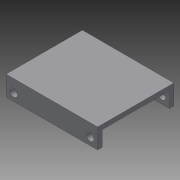
# Autodesk Inventor part: EE_Base-SquareBar-Rev3
Saved by Autodesk Inventor 2015 (Build 190159000, 159)
## iProperties
Created: 2017-01-10
Part Number: EE_Base-SquareBar-Rev3
Material: Generic
Document SubType Name: Modeling
Designer: Guy
Density: 1 g/cm^3
Appearance: Default
Author: Guy
Autodesk Inventor part; units mm, degrees
ref_plane "YZ Plane" through (0, 0, 0) normal (1, 0, 0) x (0, 1, 0)
ref_plane "XZ Plane" through (0, 0, 0) normal (0, 1, 0) x (-1, 0, 0)
ref_plane "XY Plane" through (0, 0, 0) normal (0, 0, 1) x (1, 0, 0)
sketch "Sketch1" plane through (0, 0, 0) normal (0, 0, 1) x (1, 0, 0)
  line L0 (0, 0) -> (60, 0)
  line L1 (60, 0) -> (60, 50)
  line L2 (60, 50) -> (0, 50)
  line L3 (0, 50) -> (0, 0)
  dimension "d0" = 60
  dimension "d1" = 50
  constraints: 8 end point, 2 parallel, 1 horizontal, 1 perpendicular
  measures "d0" distance of L2.end L1.end
  measures "d1" distance between parallel lines of L0 L2
extrude "Extrusion1" add sketch "Sketch1" along normal blind 3
sketch "Sketch2" plane through (0, 0, 0) normal (0, 0, -1) x (-1, 0, 0)
  line L0 (0, 0) -> (-60, 0) projected
  line L1 (0, 50) -> (0, 0) projected
  line L2 (-60, 50) -> (0, 50) projected
  line L3 (-60, 0) -> (-60, 50) projected
  line L4 (0, 0) -> (-60, 0)
  line L5 (-60, 0) -> (-60, 3)
  line L6 (-60, 3) -> (0, 3)
  line L7 (0, 3) -> (0, 0)
  line L8 (-60, 0) -> (-60, 50) projected
  line L9 (0, 50) -> (-60, 50)
  line L10 (-60, 50) -> (-60, 47)
  line L11 (-60, 47) -> (0, 47)
  line L12 (0, 47) -> (0, 50)
  dimension "d4" = 3
  dimension "d5" = 3
  constraints: 16 end point, 4 parallel, 2 horizontal, 2 perpendicular, 2 point on line
  measures "d4" distance between parallel lines of L6 L0
  measures "d5" distance between parallel lines of L2 L11
extrude "Extrusion2" add sketch "Sketch2" along normal blind 10 contours L0 L3 L6 L1 | L11 L3 L2 L1
sketch "Sketch3" plane through (0, 0, 3) normal (0, -1, 0) x (1, 0, 0)
  line L0 (60, -13) -> (60, 0) projected
  line L1 (0, 0) -> (60, 0) projected
  line L2 (0, 0) -> (0, -13) projected
  line L3 (60, -13) -> (0, -13) projected
  line L4 (60, -3) -> (0, -3) projected
  circle A0 centre (55, -8) radius 2.5
  circle A1 centre (5, -8) radius 2.5
  dimension "d8" = 5
  dimension "d9" = 5
  dimension "d10" = 5
  dimension "d11" = 5
  dimension "d12" = 5
  dimension "d13" = 5
  constraints: 2 centre point
  measures "d8" diameter of A0
  measures "d9" diameter of A1
  measures "d10" distance from line of L3 A0.centre
  measures "d11" distance from line of L3 A1.centre
  measures "d12" distance from line of L2 A1.centre
  measures "d13" distance from line of L0 A0.centre
extrude "Extrusion3" cut sketch "Sketch3" against normal through all contours A0 | A1
body "Solid1"
